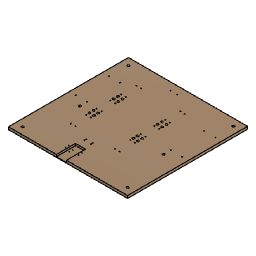
Base (Autodesk Fusion 360 design; units mm, degrees)
Autodesk Fusion 360 part; units mm, degrees
sketch "Top" plane through (0, 0, 0) normal (0, 0, 1) x (1, 0, 0)
  line L0 (420, -422.75) -> (-420, -422.75)
  line L1 (-420, -422.75) -> (-420, 422.75)
  line L2 (-420, 422.75) -> (420, 422.75)
  line L3 (420, 422.75) -> (420, -422.75)
  line L4 (420, -422.75) -> (-420, 422.75) construction
  line L5 (-420, -422.75) -> (420, 422.75) construction
  line L6 (-82, -422.75) -> (-11, -422.75)
  line L7 (-11, -422.75) -> (-11, -287.75)
  line L8 (-11, -287.75) -> (-82, -287.75)
  line L9 (-82, -287.75) -> (-82, -422.75)
  line L10 (-66.5, -323.55) -> (-26.5, -323.55) construction
  line L11 (-26.5, -323.55) -> (-26.5, -347.55) construction
  line L12 (-26.5, -347.55) -> (-66.5, -347.55) construction
  line L13 (-66.5, -347.55) -> (-66.5, -323.55) construction
  line L14 (-26.5, -323.55) -> (-11, -323.55) construction
  line L15 (-66.5, -323.55) -> (-82, -323.55) construction
  circle A0 centre (-66.5, -323.55) radius 2.5
  circle A1 centre (-26.5, -323.55) radius 2.5
  circle A2 centre (-66.5, -347.55) radius 2.5
  circle A3 centre (-26.5, -347.55) radius 2.5
  line L16 (-91.5, -320) -> (-91.5, -350) construction
  line L17 (-1.5, -320) -> (-1.5, -350) construction
  line L18 (-66.5, -347.55) -> (-91.5, -347.55) construction
  line L19 (-26.5, -347.55) -> (-1.5, -347.55) construction
  circle A4 centre (-91.5, -323.55) radius 3
  circle A5 centre (-91.5, -347.55) radius 3
  circle A6 centre (-1.5, -323.55) radius 3
  circle A7 centre (-1.5, -347.55) radius 3
  line L20 (-46.5, -323.55) -> (-46.5, -180) construction
  line L21 (-69.5, -237.75) -> (-46.5, -237.75) construction
  line L22 (-23.5, -237.75) -> (-23.5, 370.25) construction
  line L23 (-69.5, 370.25) -> (-69.5, -237.75) construction
  line L24 (-46.5, -237.75) -> (-23.5, -237.75) construction
  line L25 (-23.5, 370.25) -> (-69.5, 370.25) construction
  line L26 (-69.5, -224.75) -> (-23.5, -224.75) construction
  circle A8 centre (-69.5, -237.75) radius 3.5
  circle A9 centre (-23.5, -237.75) radius 3.5
  circle A10 centre (-69.5, -224.75) radius 3.5
  circle A11 centre (-23.5, -224.75) radius 3.5
  circle A12 centre (-23.5, 370.25) radius 3.5
  circle A13 centre (-69.5, 370.25) radius 3.5
  line L27 (91, -182.25) -> (123, -182.25) construction
  line L28 (123, -182.25) -> (123, 277.75) construction
  line L29 (123, 277.75) -> (91, 277.75) construction
  line L30 (91, 277.75) -> (91, -182.25) construction
  line L31 (91, -22.75) -> (123, -22.75) construction
  line L32 (91, -0.25) -> (123, -0.25) construction
  line L33 (91, 95.75) -> (123, 95.75) construction
  line L34 (91, 118.25) -> (123, 118.25) construction
  line L35 (91, -52.75) -> (123, -52.75) construction
  line L36 (91, -75.25) -> (123, -75.25) construction
  line L37 (123, 148.25) -> (91, 148.25) construction
  line L38 (123, 170.75) -> (91, 170.75) construction
  line L39 (-219, -75.25) -> (-187, -75.25) construction
  line L40 (-219, -52.75) -> (-187, -52.75) construction
  line L41 (-219, 95.75) -> (-187, 95.75) construction
  line L42 (-219, 277.75) -> (-219, -182.25) construction
  line L43 (-187, 170.75) -> (-219, 170.75) construction
  line L44 (-187, 277.75) -> (-219, 277.75) construction
  line L45 (-219, -182.25) -> (-187, -182.25) construction
  line L46 (-187, 148.25) -> (-219, 148.25) construction
  line L47 (-187, -182.25) -> (-187, 277.75) construction
  line L48 (-219, 118.25) -> (-187, 118.25) construction
  line L49 (-219, -0.25) -> (-187, -0.25) construction
  line L50 (-219, -22.75) -> (-187, -22.75) construction
  circle A14 centre (91, -52.75) radius 7.5
  circle A15 centre (123, -52.75) radius 7.5
  circle A16 centre (91, -22.75) radius 7.5
  circle A17 centre (123, -22.75) radius 7.5
  circle A18 centre (91, 118.25) radius 7.5
  circle A19 centre (123, 118.25) radius 7.5
  circle A20 centre (91, 148.25) radius 7.5
  circle A21 centre (123, 148.25) radius 7.5
  circle A22 centre (-219, 148.25) radius 7.5
  circle A23 centre (-187, 148.25) radius 7.5
  circle A24 centre (-219, 118.25) radius 7.5
  circle A25 centre (-187, 118.25) radius 7.5
  circle A26 centre (-219, -22.75) radius 7.5
  circle A27 centre (-187, -22.75) radius 7.5
  circle A28 centre (-219, -52.75) radius 7.5
  circle A29 centre (-187, -52.75) radius 7.5
  line L51 (-375, 240.75) -> (-295, 240.75) construction
  line L52 (-295, 240.75) -> (-295, 5.75) construction
  line L53 (-295, 5.75) -> (-375, 5.75) construction
  line L54 (-375, 5.75) -> (-375, 240.75) construction
  line L55 (295, 240.75) -> (375, 240.75) construction
  line L56 (375, 240.75) -> (375, 5.75) construction
  line L57 (375, 5.75) -> (295, 5.75) construction
  line L58 (295, 5.75) -> (295, 240.75) construction
  circle A30 centre (-375, 240.75) radius 3.5
  circle A31 centre (-295, 240.75) radius 3.5
  circle A32 centre (-375, 5.75) radius 3.5
  circle A33 centre (-295, 5.75) radius 3.5
  circle A34 centre (295, 5.75) radius 3.5
  circle A35 centre (375, 5.75) radius 3.5
  circle A36 centre (375, 240.75) radius 3.5
  circle A37 centre (295, 240.75) radius 3.5
  circle A38 centre (-219, 277.75) radius 3.5
  circle A39 centre (-219, 277.75) radius 7.5
  circle A40 centre (-187, 277.75) radius 3.5
  circle A41 centre (-187, 277.75) radius 7.5
  circle A42 centre (-219, 170.75) radius 3.5
  circle A43 centre (-219, 170.75) radius 7.5
  circle A44 centre (-187, 170.75) radius 3.5
  circle A45 centre (-187, 170.75) radius 7.5
  circle A46 centre (91, 277.75) radius 3.5
  circle A47 centre (91, 277.75) radius 7.5
  circle A48 centre (123, 277.75) radius 3.5
  circle A49 centre (123, 277.75) radius 7.5
  circle A50 centre (91, 170.75) radius 3.5
  circle A51 centre (91, 170.75) radius 7.5
  circle A52 centre (123, 170.75) radius 3.5
  circle A53 centre (123, 170.75) radius 7.5
  circle A54 centre (91, 95.75) radius 3.5
  circle A55 centre (91, 95.75) radius 7.5
  circle A56 centre (123, 95.75) radius 3.5
  circle A57 centre (123, 95.75) radius 7.5
  circle A58 centre (-219, 95.75) radius 3.5
  circle A59 centre (-219, 95.75) radius 7.5
  circle A60 centre (-187, 95.75) radius 3.5
  circle A61 centre (-187, 95.75) radius 7.5
  circle A62 centre (-219, -0.25) radius 3.5
  circle A63 centre (-219, -0.25) radius 7.5
  circle A64 centre (-187, -0.25) radius 3.5
  circle A65 centre (-187, -0.25) radius 7.5
  circle A66 centre (-219, -75.25) radius 3.5
  circle A67 centre (-219, -75.25) radius 7.5
  circle A68 centre (-187, -75.25) radius 3.5
  circle A69 centre (-187, -75.25) radius 7.5
  circle A70 centre (91, -0.25) radius 3.5
  circle A71 centre (91, -0.25) radius 7.5
  circle A72 centre (123, -0.25) radius 3.5
  circle A73 centre (123, -0.25) radius 7.5
  circle A74 centre (91, -75.25) radius 3.5
  circle A75 centre (91, -75.25) radius 7.5
  circle A76 centre (123, -75.25) radius 3.5
  circle A77 centre (123, -75.25) radius 7.5
  circle A78 centre (91, -182.25) radius 3.5
  circle A79 centre (91, -182.25) radius 7.5
  circle A80 centre (123, -182.25) radius 3.5
  circle A81 centre (123, -182.25) radius 7.5
  circle A82 centre (-219, -182.25) radius 3.5
  circle A83 centre (-219, -182.25) radius 7.5
  circle A84 centre (-187, -182.25) radius 3.5
  circle A85 centre (-187, -182.25) radius 7.5
  circle A86 centre (-370, -372.75) radius 3
  circle A87 centre (370, -372.75) radius 3
  circle A88 centre (370, 372.75) radius 3
  circle A89 centre (-370, 372.75) radius 3
  circle A90 centre (-295, -44.25) radius 3
  circle A91 centre (295, -44.25) radius 3
  dimension "d1" = 845.5
  dimension "d2" = 840
  dimension "d3" = 71
  dimension "d4" = 135
  dimension "d6" = 40
  dimension "d7" = 24
  dimension "d9" = 5
  dimension "d10" = 5
  dimension "d11" = 5
  dimension "d12" = 5
  dimension "d14" = 90
  dimension "d15" = 6
  dimension "d16" = 6
  dimension "d17" = 6
  dimension "d18" = 6
  dimension "d23" = 13
  dimension "d24" = 608
  dimension "d25" = 46
  dimension "d26" = 185
  dimension "d27" = 7
  dimension "d28" = 7
  dimension "d29" = 7
  dimension "d30" = 7
  dimension "d31" = 7
  dimension "d32" = 7
  dimension "d33" = 32
  dimension "d34" = 460
  dimension "d35" = 107
  dimension "d36" = 107
  dimension "d37" = 22.5
  dimension "d38" = 30
  dimension "d39" = 22.5
  dimension "d40" = 22.5
  dimension "d41" = 30
  dimension "d42" = 22.5
  dimension "d43" = 116
  dimension "d44" = 32
  dimension "d45" = 460
  dimension "d46" = 107
  dimension "d47" = 107
  dimension "d48" = 22.5
  dimension "d49" = 30
  dimension "d50" = 22.5
  dimension "d51" = 22.5
  dimension "d52" = 30
  dimension "d53" = 22.5
  dimension "d54" = 278
  dimension "d55" = 114.5
  dimension "d56" = 240.5
  dimension "d61" = 15
  dimension "d62" = 15
  dimension "d63" = 15
  dimension "d64" = 15
  dimension "d69" = 15
  dimension "d70" = 15
  dimension "d71" = 15
  dimension "d72" = 15
  dimension "d81" = 15
  dimension "d82" = 15
  dimension "d83" = 15
  dimension "d84" = 15
  dimension "d89" = 15
  dimension "d90" = 15
  dimension "d91" = 15
  dimension "d92" = 15
  dimension "d97" = 80
  dimension "d98" = 235
  dimension "d99" = 80
  dimension "d100" = 235
  dimension "d101" = 7
  dimension "d102" = 7
  dimension "d103" = 7
  dimension "d104" = 7
  dimension "d105" = 7
  dimension "d106" = 7
  dimension "d107" = 7
  dimension "d108" = 7
  dimension "d109" = 45
  dimension "d110" = 45
  dimension "d111" = 182
  dimension "d112" = 182
  dimension "d155" = 466.5
  dimension "d156" = 75.2
  dimension "d158" = 240
  dimension "d159" = 258
  dimension "d182" = 7
  dimension "d183" = 15
  dimension "d184" = 7
  dimension "d185" = 15
  dimension "d186" = 7
  dimension "d187" = 15
  dimension "d188" = 7
  dimension "d189" = 15
  dimension "d190" = 7
  dimension "d191" = 15
  dimension "d192" = 7
  dimension "d193" = 15
  dimension "d194" = 7
  dimension "d195" = 15
  dimension "d196" = 7
  dimension "d197" = 15
  dimension "d198" = 7
  dimension "d199" = 15
  dimension "d200" = 7
  dimension "d201" = 15
  dimension "d202" = 7
  dimension "d203" = 15
  dimension "d204" = 7
  dimension "d205" = 15
  dimension "d206" = 7
  dimension "d207" = 15
  dimension "d208" = 7
  dimension "d209" = 15
  dimension "d210" = 7
  dimension "d211" = 15
  dimension "d212" = 7
  dimension "d213" = 15
  dimension "d214" = 7
  dimension "d215" = 15
  dimension "d216" = 7
  dimension "d217" = 15
  dimension "d218" = 7
  dimension "d219" = 15
  dimension "d220" = 7
  dimension "d221" = 15
  dimension "d222" = 7
  dimension "d223" = 15
  dimension "d224" = 7
  dimension "d225" = 15
  dimension "d226" = 7
  dimension "d227" = 15
  dimension "d228" = 7
  dimension "d229" = 15
  dimension "d235" = 6
  dimension "d236" = 50
  dimension "d237" = 50
  dimension "d238" = 6
  dimension "d239" = 6
  dimension "d240" = 6
  dimension "d241" = 6
  dimension "d242" = 6
  dimension "d243" = 50
  dimension "d244" = 50
  dimension "d245" = 50
  dimension "d246" = 50
  dimension "d247" = 50
  dimension "d248" = 50
  dimension "d249" = 50
  dimension "d250" = 50
  constraint perpendicular L0 L1
  constraint parallel L0 L2
  constraint parallel L1 L3
  constraint horizontal L0
  constraint coincident L4 origin
  constraint coincident L5 origin
  constraint horizontal L6
  constraint vertical L7
  constraint horizontal L8
  constraint vertical L9
  constraint coincident L0 L6.start
  constraint horizontal L10
  constraint vertical L11
  constraint horizontal L12
  constraint vertical L13
  constraint coincident L7 L14.end
  constraint perpendicular L7 L14
  constraint coincident L9 L15.end
  constraint perpendicular L9 L15
  constraint equal L14 L15
  constraint coincident L10.start L13.end
  constraint coincident L10.end L11.start
  constraint coincident L12.end L13.start
  constraint coincident L11.end L12.start
  constraint perpendicular L15 L16
  constraint perpendicular L14 L17
  constraint coincident L16 L18.end
  constraint perpendicular L16 L18
  constraint coincident L17 L19.end
  constraint perpendicular L17 L19
  constraint equal L18 L19
  constraint coincident L16 A4.centre
  constraint coincident L18.end A5.centre
  constraint coincident L17 A6.centre
  constraint coincident L19.end A7.centre
  constraint midpoint L10 L20.start
  constraint perpendicular L8 L20
  constraint coincident L20 L21.end
  constraint perpendicular L20 L21
  constraint perpendicular L21 L23
  constraint perpendicular L22 L24
  constraint collinear L21 L24
  constraint equal L21 L24
  constraint perpendicular L23 L25
  constraint coincident L23 L26.start
  constraint coincident L22 L26.end
  constraint perpendicular L22 L26
  constraint coincident L21.start L23.end
  constraint coincident L22.start L24.end
  constraint coincident L26.start A10.centre
  constraint coincident L26.end A11.centre
  constraint coincident L22.end L25.start
  constraint coincident L23.start L25.end
  constraint horizontal L27
  constraint vertical L28
  constraint horizontal L29
  constraint vertical L30
  constraint coincident L30 L31.start
  constraint coincident L28 L31.end
  constraint perpendicular L28 L31
  constraint coincident L30 L32.start
  constraint coincident L28 L32.end
  constraint perpendicular L28 L32
  constraint coincident L30 L33.start
  constraint coincident L28 L33.end
  constraint perpendicular L28 L33
  constraint coincident L30 L34.start
  constraint coincident L28 L34.end
  constraint perpendicular L28 L34
  constraint coincident L30 L35.start
  constraint coincident L28 L35.end
  constraint perpendicular L28 L35
  constraint coincident L30 L36.start
  constraint perpendicular L30 L36
  constraint coincident L28 L36.end
  constraint coincident L28 L37.start
  constraint perpendicular L28 L37
  constraint coincident L30 L37.end
  constraint coincident L28 L38.start
  constraint perpendicular L28 L38
  constraint coincident L30 L38.end
  constraint horizontal L45
  constraint vertical L47
  constraint horizontal L44
  constraint vertical L42
  constraint coincident L50.start L42
  constraint coincident L50.end L47
  constraint perpendicular L47 L50
  constraint coincident L49.start L42
  constraint coincident L49.end L47
  constraint perpendicular L47 L49
  constraint coincident L41.start L42
  constraint coincident L41.end L47
  constraint perpendicular L41 L47
  constraint coincident L48.start L42
  constraint coincident L48.end L47
  constraint perpendicular L47 L48
  constraint coincident L40.start L42
  constraint coincident L40.end L47
  constraint perpendicular L40 L47
  constraint coincident L39.start L42
  constraint perpendicular L39 L42
  constraint coincident L39.end L47
  constraint coincident L46.start L47
  constraint perpendicular L46 L47
  constraint coincident L46.end L42
  constraint coincident L43.start L47
  constraint perpendicular L43 L47
  constraint coincident L43.end L42
  constraint collinear L27 L45
  constraint coincident L35.start A14.centre
  constraint coincident L35.end A15.centre
  constraint coincident L31.start A16.centre
  constraint coincident L31.end A17.centre
  constraint coincident L34.start A18.centre
  constraint coincident L34.end A19.centre
  constraint coincident L37.end A20.centre
  constraint coincident L37.start A21.centre
  constraint coincident L46.end A22.centre
  constraint coincident L46.start A23.centre
  constraint coincident L48.start A24.centre
  constraint coincident L48.end A25.centre
  constraint coincident L50.start A26.centre
  constraint coincident L50.end A27.centre
  constraint coincident L40.start A28.centre
  constraint coincident L40.end A29.centre
  constraint horizontal L51
  constraint vertical L52
  constraint horizontal L53
  constraint vertical L54
  constraint horizontal L55
  constraint vertical L56
  constraint horizontal L57
  constraint vertical L58
  constraint coincident L51.start L54.end
  constraint coincident L51.end L52.start
  constraint coincident L53.end L54.start
  constraint coincident L52.end L53.start
  constraint coincident L57.end L58.start
  constraint coincident L56.end L57.start
  constraint coincident L55.end L56.start
  constraint coincident L55.start L58.end
  constraint coincident L42.start L44.end
  constraint concentric A38 A39
  constraint coincident L44.start L47.end
  constraint concentric A40 A41
  constraint coincident L43.end A42.centre
  constraint concentric A42 A43
  constraint coincident L43.start A44.centre
  constraint concentric A44 A45
  constraint coincident L29.end L30.start
  constraint concentric A46 A47
  constraint coincident L28.end L29.start
  constraint concentric A48 A49
  constraint coincident L38.end A50.centre
  constraint concentric A50 A51
  constraint coincident L38.start A52.centre
  constraint concentric A52 A53
  constraint coincident L33.start A54.centre
  constraint concentric A54 A55
  constraint coincident L33.end A56.centre
  constraint concentric A56 A57
  constraint coincident L41.start A58.centre
  constraint concentric A58 A59
  constraint coincident L41.end A60.centre
  constraint concentric A60 A61
  constraint coincident L49.start A62.centre
  constraint concentric A62 A63
  constraint coincident L49.end A64.centre
  constraint concentric A64 A65
  constraint coincident L39.start A66.centre
  constraint concentric A66 A67
  constraint coincident L39.end A68.centre
  constraint concentric A68 A69
  constraint coincident L32.start A70.centre
  constraint concentric A70 A71
  constraint coincident L32.end A72.centre
  constraint concentric A72 A73
  constraint coincident L36.start A74.centre
  constraint concentric A74 A75
  constraint coincident L36.end A76.centre
  constraint concentric A76 A77
  constraint coincident L27.start L30.end
  constraint concentric A78 A79
  constraint coincident L27.end L28.start
  constraint concentric A80 A81
  constraint coincident L42.end L45.start
  constraint concentric A82 A83
  constraint coincident L45.end L47.start
  constraint concentric A84 A85
  measures "d1" distance of L0.end L1.end
  measures "d2" distance of L1.end L2.end
  measures "d3" distance of L6.start L6.end
  measures "d4" distance of L6.start L8.end
  measures "d6" distance of L10.start L10.end
  measures "d7" distance of L10.start L12.end
  measures "d9" diameter of A0
  measures "d10" diameter of A1
  measures "d11" diameter of A2
  measures "d12" diameter of A3
  measures "d14" distance of L16 L17
  measures "d15" diameter of A4
  measures "d16" diameter of A5
  measures "d17" diameter of A6
  measures "d18" diameter of A7
  measures "d23" distance of L24 L26
  measures "d24" distance of L21 L25
  measures "d25" distance of L22.end L23.start
  measures "d26" distance of L0 L24
  measures "d27" diameter of A8
  measures "d28" diameter of A9
  measures "d29" diameter of A10
  measures "d30" diameter of A11
  measures "d31" diameter of A12
  measures "d32" diameter of A13
  measures "d33" distance of L27.start L27.end
  measures "d34" distance of L27.start L29.end
  measures "d35" distance of L27 L36
  measures "d36" distance of L29 L38
  measures "d37" distance of L37 L38
  measures "d38" distance of L34 L37
  measures "d39" distance of L33 L34
  measures "d40" distance of L31 L32
  measures "d41" distance of L31 L35
  measures "d42" distance of L35 L36
  measures "d44" distance of L42.end L45.end
  measures "d45" distance of L42.end L42.start
  measures "d46" distance of L39 L45
  measures "d47" distance of L43 L44
  measures "d48" distance of L43 L46
  measures "d49" distance of L46 L48
  measures "d50" distance of L41 L48
  measures "d51" distance of L49 L50
  measures "d52" distance of L40 L50
  measures "d53" distance of L39 L40
  measures "d54" distance of L30 L47
  measures "d55" distance of L26.end L30
  measures "d56" distance of L0 L27
  measures "d61" diameter of A14
  measures "d62" diameter of A15
  measures "d63" diameter of A16
  measures "d64" diameter of A17
  measures "d69" diameter of A18
  measures "d70" diameter of A19
  measures "d71" diameter of A20
  measures "d72" diameter of A21
  measures "d81" diameter of A22
  measures "d82" diameter of A23
  measures "d83" diameter of A24
  measures "d84" diameter of A25
  measures "d89" diameter of A26
  measures "d90" diameter of A27
  measures "d91" diameter of A28
  measures "d92" diameter of A29
  measures "d97" distance of L51.start L51.end
  measures "d98" distance of L51.start L53.end
  measures "d99" distance of L55.start L55.end
  measures "d100" distance of L55.start L57.end
  measures "d101" diameter of A30
  measures "d102" diameter of A31
  measures "d103" diameter of A32
  measures "d104" diameter of A33
  measures "d105" diameter of A34
  measures "d106" diameter of A35
  measures "d107" diameter of A36
  measures "d108" diameter of A37
  measures "d109" distance of L1 L54
  measures "d110" distance of L3 L56
  measures "d111" distance of L2 L55
  measures "d112" distance of L2 L51
  measures "d155" distance of L3 L20
  measures "d156" distance of L6 L12
  measures "d182" diameter of A38
  measures "d183" diameter of A39
  measures "d184" diameter of A40
  measures "d185" diameter of A41
  measures "d186" diameter of A42
  measures "d187" diameter of A43
  measures "d188" diameter of A44
  measures "d189" diameter of A45
  measures "d190" diameter of A46
  measures "d191" diameter of A47
  measures "d192" diameter of A48
  measures "d193" diameter of A49
  measures "d194" diameter of A50
  measures "d195" diameter of A51
  measures "d196" diameter of A52
  measures "d197" diameter of A53
  measures "d198" diameter of A54
  measures "d199" diameter of A55
  measures "d200" diameter of A56
  measures "d201" diameter of A57
  measures "d202" diameter of A58
  measures "d203" diameter of A59
  measures "d204" diameter of A60
  measures "d205" diameter of A61
  measures "d206" diameter of A62
  measures "d207" diameter of A63
  measures "d208" diameter of A64
  measures "d209" diameter of A65
  measures "d210" diameter of A66
  measures "d211" diameter of A67
  measures "d212" diameter of A68
  measures "d213" diameter of A69
  measures "d214" diameter of A70
  measures "d215" diameter of A71
  measures "d216" diameter of A72
  measures "d217" diameter of A73
  measures "d218" diameter of A74
  measures "d219" diameter of A75
  measures "d220" diameter of A76
  measures "d221" diameter of A77
  measures "d222" diameter of A78
  measures "d223" diameter of A79
  measures "d224" diameter of A80
  measures "d225" diameter of A81
  measures "d226" diameter of A82
  measures "d227" diameter of A83
  measures "d228" diameter of A84
  measures "d229" diameter of A85
  measures "d235" diameter of A86
  measures "d236" distance of L0 A86.centre
  measures "d237" distance of L1 A86.centre
  measures "d238" diameter of A87
  measures "d239" diameter of A88
  measures "d240" diameter of A89
  measures "d241" diameter of A90
  measures "d242" diameter of A91
  measures "d243" distance of L0 A87.centre
  measures "d244" distance of L3 A87.centre
  measures "d245" distance of L2 A88.centre
  measures "d246" distance of L3 A88.centre
  measures "d247" distance of L2 A89.centre
  measures "d248" distance of L1 A89.centre
  measures "d249" distance of L52.end A90.centre
  measures "d250" distance of L57.end A91.centre
extrude "Extrude1" add sketch "Top" along normal blind 18 contours L0 L1 L2 L3 L7 L8 L9
extrude "Extrude11" add sketch "Top" along normal blind 4 contours L0 L6 L7 L8 L9
extrude "Extrude12" add sketch "Top" along normal blind 9 from surface at 9 contours A39 | A41 | A43 | A45 | A47 | A49 | A51 | A53 | A55 | A57 | A59 | A61 | A63 | A65 | A67 | A69 | A71 | A73 | A75 | A77 | A79 | A81 | A83 | A85
chamfer "Chamfer1" distance 5 angle 45 6 edges at (-372.797, -371.6652, 18) (-297.797, -43.1652, 18) (-372.797, 373.8348, 18) (367.203, 373.8348, 18) (292.203, -43.1652, 18) (367.203, -371.6652, 18)
equation "d61 = M6WasherClearance"
equation "d62 = M6WasherClearance"
equation "d63 = M6WasherClearance"
equation "d64 = M6WasherClearance"
equation "d69 = M6WasherClearance"
equation "d70 = M6WasherClearance"
equation "d71 = M6WasherClearance"
equation "d72 = M6WasherClearance"
equation "d81 = M6WasherClearance"
equation "d82 = M6WasherClearance"
equation "d83 = M6WasherClearance"
equation "d84 = M6WasherClearance"
equation "d89 = M6WasherClearance"
equation "d90 = M6WasherClearance"
equation "d91 = M6WasherClearance"
equation "d92 = M6WasherClearance"
equation "M6WasherClearance = 15 mm"
equation "M5ClearHole = 6 mm"
equation "M6ClearHole = 7 mm"
equation "d182 = M6ClearHole"
equation "d183 = M6WasherClearance"
equation "d184 = M6ClearHole"
equation "d185 = M6WasherClearance"
equation "d186 = M6ClearHole"
equation "d187 = M6WasherClearance"
equation "d188 = M6ClearHole"
equation "d189 = M6WasherClearance"
equation "d190 = M6ClearHole"
equation "d191 = M6WasherClearance"
equation "d192 = M6ClearHole"
equation "d193 = M6WasherClearance"
equation "d194 = M6ClearHole"
equation "d195 = M6WasherClearance"
equation "d196 = M6ClearHole"
equation "d197 = M6WasherClearance"
equation "d198 = M6ClearHole"
equation "d199 = M6WasherClearance"
equation "d200 = M6ClearHole"
equation "d201 = M6WasherClearance"
equation "d202 = M6ClearHole"
equation "d203 = M6WasherClearance"
equation "d204 = M6ClearHole"
equation "d205 = M6WasherClearance"
equation "d206 = M6ClearHole"
equation "d207 = M6WasherClearance"
equation "d208 = M6ClearHole"
equation "d209 = M6WasherClearance"
equation "d210 = M6ClearHole"
equation "d211 = M6WasherClearance"
equation "d212 = M6ClearHole"
equation "d213 = M6WasherClearance"
equation "d214 = M6ClearHole"
equation "d215 = M6WasherClearance"
equation "d216 = M6ClearHole"
equation "d217 = M6WasherClearance"
equation "d218 = M6ClearHole"
equation "d219 = M6WasherClearance"
equation "d220 = M6ClearHole"
equation "d221 = M6WasherClearance"
equation "d222 = M6ClearHole"
equation "d223 = M6WasherClearance"
equation "d224 = M6ClearHole"
equation "d225 = M6WasherClearance"
equation "d226 = M6ClearHole"
equation "d227 = M6WasherClearance"
equation "d228 = M6ClearHole"
equation "d229 = M6WasherClearance"
equation "d243 = d236"
equation "d244 = d237"
equation "d245 = d236"
equation "d246 = d237"
equation "d247 = d236"
equation "d248 = d237"
equation "d249 = d236"
equation "d250 = d236"
named bodies: "Base"
